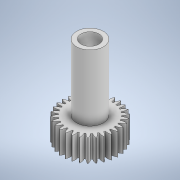
# Autodesk Inventor part: Skrzynia-srodek-zebatka
Saved by Autodesk Inventor 2022 (Build 260153000, 153)
## iProperties
Created: 2022-03-27
Part Number: Skrzynia-srodek-zebatka
Material: Ogólny
Document SubType Name: Modeling
Designer: jolow
Density: 1 g/cm^3
Appearance: Domyślna
Author: jolow
Autodesk Inventor part; units mm, degrees
ref_plane "YZ Plane" through (0, 0, 0) normal (1, 0, 0) x (0, 1, 0)
ref_plane "XZ Plane" through (0, 0, 0) normal (0, 1, 0) x (-1, 0, 0)
ref_plane "XY Plane" through (0, 0, 0) normal (0, 0, 1) x (1, 0, 0)
sketch "Szkic1" plane through (0, 0, 0) normal (0, 1, 0) x (-1, 0, 0)
  circle A0 centre (0, 0) radius 20
  dimension "d0" = 40
  constraints: 1 centre point, 1 coincident
  measures "d0" diameter of A0
extrude "Wyciągnięcie proste1" add sketch "Szkic1" along normal blind 20
sketch "Szkic2" plane through (0, 0, 0) normal (0, -1, 0) x (-1, 0, 0)
  circle A0 centre (0, 0) radius 20 projected
  line L0 (25.0437, -0.1347) -> (25.0437, 0.1393)
  line L1 (19.9437, 1.5) -> (19.9437, -1.5)
  arc A1 (24.9034, 0.1192) -> (19.9437, 1.5) centre (20.1106, -7.4985) ccw
  arc A2 (19.9437, -1.5) -> (24.9037, -0.1144) centre (20.1035, 7.4986) ccw
  arc A3 (25.0437, -0.1347) -> (24.9034, 0.1192) centre (24.7437, -0.1347) ccw
  arc A4 (24.9037, -0.1144) -> (25.0437, 0.1393) centre (24.7437, 0.1393) ccw
  point P0 (25.0437, 0.0292)
  point P1 (25.0437, -0.0244)
  point P2 (25.0105, 0.0023)
  dimension "d6" = 9
  dimension "d5" = 9
  dimension "d4" = 0.3
  dimension "d7" = 3
  constraints: 12 point on circle, 4 centre point, 4 end point, 4 tangent, 2 point on line, 1 equal radius, 1 parallel, 1 vertical
  measures "d6" radius of A1
  measures "d5" radius of A2
  measures "d4" radius of A3
  measures "d7" distance of L1.start L1.end
extrude "Wyciągnięcie proste2" add sketch "Szkic2" against normal blind 20 contours A0 A1 A3 A4 A2
pattern_circular "Szyk kołowy1" count 30 over 360 about axis through (0, 0, 0) along (0, 1, 0) of "Wyciągnięcie proste2"
sketch "Szkic3" plane through (0, 20, 0) normal (0, 1, 0) x (1, 0, 0)
  circle A0 centre (0, 0) radius 12
  circle A1 centre (0, 0) radius 8
  dimension "d15" = 24
  dimension "d16" = 16
  dimension "d21" = 4
  constraints: 2 centre point, 2 coincident
  measures "d15" diameter of A0
  measures "d16" diameter of A1
  measures "d21" radial gap between concentric circles of A0 A1
extrude "Wyciągnięcie proste3" add sketch "Szkic3" along normal blind 59
sketch "Szkic4" plane through (0, 20, 0) normal (0, 1, 0) x (1, 0, 0)
  circle A0 centre (0, 0) radius 7.5
  constraints: 1 centre point, 1 coincident
extrude "Wyciągnięcie proste4" cut sketch "Szkic4" against normal through all
